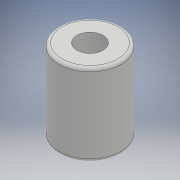
# Autodesk Inventor part: Acoplamento5Para8
Saved by Autodesk Inventor 2018 (Build 220112000, 112)
## iProperties
Created: 2018-09-20
Part Number: Acoplamento5Para8
Material: Genérico
Document SubType Name: Modeling
Designer: Georgines
Density: 1 g/cm^3
Appearance: Padrão
Author: Georgines
Autodesk Inventor part; units mm, degrees
ref_plane "YZ Plane" through (0, 0, 0) normal (1, 0, 0) x (0, 1, 0)
ref_plane "XZ Plane" through (0, 0, 0) normal (0, 1, 0) x (-1, 0, 0)
ref_plane "XY Plane" through (0, 0, 0) normal (0, 0, 1) x (1, 0, 0)
sketch "Esboço1" plane through (0, 0, 0) normal (0, 0, 1) x (1, 0, 0)
  circle A0 centre (0, 0) radius 9.5
  dimension "d0" = 19
  constraints: 1 centre point, 1 coincident
  measures "d0" diameter of A0
extrude "Extrusão1" add sketch "Esboço1" along normal blind 25
sketch "Esboço4" plane through (0, 0, 25) normal (0, 0, 1) x (1, 0, 0)
  circle A0 centre (0, 0) radius 1.7116
  constraints: 1 centre point, 1 coincident
hole "Furo1" at (0, 0, 25) direction (0, 0, -1) diameter 5 end through all counterbore diameter 8 counterbore depth 9.5
fillet "Arredondamento1" radius 1 2 edges at (-9.5, 0, 0) (-9.5, 0, 25)
